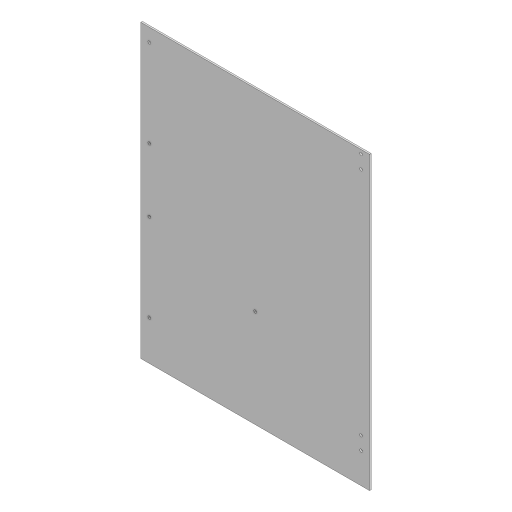
# Autodesk Inventor part: front_door
Saved by Autodesk Inventor 2023 (Build 270158000, 158)
## iProperties
Created: 2024-06-05
Part Number: front_door
Material: Generic
Document SubType Name: Modeling
Designer: nvladi
Density: 1 g/cm^3
Appearance: Default
Author: nvladi
Autodesk Inventor part; units mm, degrees
ref_plane "YZ Plane" through (0, 0, 0) normal (1, 0, 0) x (0, 1, 0)
ref_plane "XZ Plane" through (0, 0, 0) normal (0, 1, 0) x (-1, 0, 0)
ref_plane "XY Plane" through (0, 0, 0) normal (0, 0, 1) x (1, 0, 0)
sketch "Sketch1" plane through (0, 0, 0) normal (0, 0, 1) x (1, 0, 0)
  line L0 (0, 0) -> (432, 0)
  line L1 (432, 0) -> (432, 550)
  line L2 (432, 550) -> (0, 550)
  line L3 (0, 550) -> (0, 0)
  line L4 (26.4098, 50) -> (392.639, 50) construction
  line L5 (16, 512.9511) -> (16, 47.9511) construction
  line L6 (416, 495.7619) -> (416, 50) construction
  point P0 (416, 542.5)
  point P1 (416, 517.5)
  point P2 (416, 82.5)
  point P3 (416, 57.5)
  point P4 (16, 360)
  point P5 (16, 240)
  point P6 (216, 185)
  point P7 (16, 525)
  point P8 (16, 75)
  dimension "d0" = 432
  dimension "d1" = 550
  dimension "d2" = 7.5
  dimension "d3" = 25
  dimension "d5" = 25
  dimension "d7" = 120
  dimension "d8" = 190
  dimension "d10" = 500
  dimension "d11" = 135
  dimension "d12" = 200
  dimension "d13" = 25
  dimension "d14" = 25
  dimension "d15" = 16
  dimension "d16" = 16
  dimension "d26" = 7.5
  constraints: 14 end point, 5 vertical alignment, 3 parallel, 3 point on line, 2 horizontal, 1 perpendicular, 1 vertical
  measures "d0" distance of L2.end L1.end
  measures "d1" distance of L1.end L0.end
  measures "d2" distance from line of point (416, 542.5) L2
  measures "d3" distance of point (416, 517.5) point (416, 542.5)
  measures "d5" distance of point (416, 57.5) point (416, 82.5)
  measures "d7" distance of point (16, 240) point (16, 360)
  measures "d8" distance from line of point (16, 360) L2
  measures "d10" distance between parallel lines of L4 L2
  measures "d11" distance from line of L4 point (216, 185)
  measures "d12" distance from line of L5 point (216, 185)
  measures "d13" distance from line of point (16, 525) L2
  measures "d14" distance from line of L4 point (16, 75)
  measures "d15" distance between parallel lines of L3 L5
  measures "d16" distance between parallel lines of L1 L6
  measures "d26" vertical distance of L4.end point (416, 57.5)
extrude "Extrusion1" add sketch "Sketch1" along normal blind 3
hole "Hole1" at (416, 542.5, 0) at (416, 517.5, 0) at (416, 82.5, 0) at (416, 57.5, 0) at (16, 360, 0) at (16, 240, 0) at (216, 185, 0) at (16, 525, 0) at (16, 75, 0) direction (0, 0, 1) diameter 5.3 end through all
body "Solid1"
